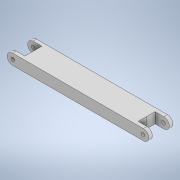
# Autodesk Inventor part: supportPiece
Saved by Autodesk Inventor 2020.3 (Build 243373000, 373)
## iProperties
Created: 2020-05-27
Part Number: supportPiece
Material: Generic
Document SubType Name: Modeling
Designer: robst
Density: 1 g/cm^3
Appearance: Default
Author: robst
Autodesk Inventor part; units mm, degrees
ref_plane "YZ Plane" through (0, 0, 0) normal (1, 0, 0) x (0, 1, 0)
ref_plane "XZ Plane" through (0, 0, 0) normal (0, 1, 0) x (-1, 0, 0)
ref_plane "XY Plane" through (0, 0, 0) normal (0, 0, 1) x (1, 0, 0)
sketch "Sketch1" plane through (0, 0, 0) normal (0, 1, 0) x (-1, 0, 0)
  line L0 (63.5003, 10.795) -> (-63.5003, 10.795)
  line L1 (-63.5, -10.795) -> (63.5, -10.795)
  line L2 (63.5003, 10.795) -> (-63.5, -10.795) construction
  line L3 (-63.5003, 10.795) -> (63.5, -10.795) construction
  line L4 (-63.5, -7.62) -> (-50.8, -7.62)
  line L5 (-50.8, -7.62) -> (-50.8, 0)
  line L6 (0, 0) -> (-63.5, -0.0014) construction
  line L7 (0, 0) -> (0, -10.795) construction
  line L8 (-63.5003, 7.6171) -> (-50.8003, 7.6177)
  line L9 (-50.8003, 7.6177) -> (-50.8, 0)
  line L10 (63.5, -7.62) -> (50.8, -7.62)
  line L11 (50.8, -7.62) -> (50.8, 0)
  line L12 (63.5003, 7.6171) -> (50.8003, 7.6177)
  line L13 (50.8003, 7.6177) -> (50.8, 0)
  line L14 (63.5, -10.795) -> (63.5, -7.62)
  line L15 (63.5003, 7.6171) -> (63.5003, 10.795)
  line L16 (-63.5003, 10.795) -> (-63.5003, 7.6171)
  line L17 (-63.5, -7.62) -> (-63.5, -10.795)
  dimension "length" = 127
  dimension "oneHalfCutoffWidth" = 7.62
  dimension "cutoutWidth" = 12.7
  dimension "width" = 21.59
  constraints: 36 end point, 7 symmetric about line, 6 parallel, 2 perpendicular, 2 point on line, 1 horizontal, 1 midpoint, 1 vertical
  measures "length" distance of L1.start L1.end
  measures "oneHalfCutoffWidth" distance from line of L4 L6.start
  measures "cutoutWidth" distance of L4.start L4.end
  measures "width" distance from line of L0 L7.end
extrude "Extrusion1" add sketch "Sketch1" along normal mid plane 9.525
sketch "Sketch2" plane through (-63.5003, 4.7625, 10.795) normal (0, 0, 1) x (1, 0, 0)
  line L0 (63.5003, -4.7625) -> (63.5003, 0) construction
  line L1 (0, 0) -> (127.0007, 0) construction
  point P0 (121.9203, -4.7625)
  point P1 (5.0803, -4.7625)
  dimension "d8" = 58.42
  constraints: 2 end point, 1 midpoint, 1 symmetric about line
  measures "d8" distance of point (121.92, -4.763) L0.start
hole "Hole1" at (58.42, 0, 10.795) at (-58.42, 0, 10.795) direction (0, 0, -1) diameter 3.2766 end through all clearance for "Flat Head Machine Screw (82)" size "#4" standard "Ansi Unified Screw Threads"
fillet "Fillet2" radius 4.7625 8 edges at (63.5, 4.7625, -9.2075) (63.5, -4.7625, -9.2075) (63.5003, 4.7625, 9.2061) (63.5003, -4.7625, 9.2061) (-63.5003, 4.7625, 9.2061) (-63.5003, -4.7625, 9.2061) (-63.5, 4.7625, -9.2075) (-63.5, -4.7625, -9.2075)
equation "\"endFilet\" = 0.5 * depth"
equation "\"depth\" = 9.525"
body "Solid1"
